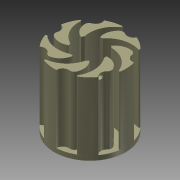
# Autodesk Inventor part: mecanum adapter
Saved by Autodesk Inventor 2015 (Build 190159000, 159)
## iProperties
Created: 2015-06-15
Part Number: mecanum adapter
Material: PBT Plastic
Document SubType Name: Modeling
Designer: Eduardo
Density: 1.31 g/cm^3
Appearance: Smooth - Ash
Author: Eduardo
Autodesk Inventor part; units mm, degrees
sketch "Sketch1" plane through (0, 0, 0) normal (0, 1, 0) x (-1, 0, 0)
  circle A0 centre (-2, -1.4) radius 8.6
  spline S0 degree 3 poles (5.001344, -1.681513) (4.992875, -1.892141) (4.974942, -2.101855) (4.947573, -2.310661) (4.933888, -2.415064) (4.917836, -2.519239) (4.89941, -2.623185) (4.880984, -2.727131) (4.858346, -2.840009) (4.833661, -2.948917) (4.734921, -3.384548) (4.597962, -3.804345) (4.410014, -4.230097) (4.222066, -4.655849) (3.994283, -5.059483) (3.719702, -5.447551) (3.445121, -5.83562) (3.130869, -6.195565) (2.783456, -6.52018) (2.522897, -6.76364) (2.245078, -6.986153) (1.949885, -7.187605) (1.851487, -7.254756) (1.752962, -7.318352) (1.653634, -7.379049) (1.355648, -7.561141) (1.045536, -7.720218) (0.723215, -7.856172) (0.669495, -7.878831) (0.613897, -7.901438) (0.561796, -7.921904) (0.171037, -8.075397) (-0.230384, -8.192863) (-0.642498, -8.274244) (-0.669972, -8.279669) (-0.699102, -8.285231) (-0.725059, -8.290035) (-0.776973, -8.299642) (-0.828947, -8.308653) (-0.88098, -8.317071) (-1.297249, -8.384413) (-1.719077, -8.414013) (-2.140737, -8.405573) (-2.351568, -8.401353) (-2.56161, -8.387632) (-2.770875, -8.364469) (-2.980139, -8.341306) (-3.18411, -8.309825) (-3.403209, -8.265052) (-3.622307, -8.220279) (-3.838521, -8.165183) (-4.051879, -8.099841) (-4.265237, -8.034498) (-4.472115, -7.96054) (-4.687338, -7.871176) (-4.902561, -7.781811) (-5.112501, -7.682071) (-5.31721, -7.572049) (-5.521919, -7.462027) (-5.719614, -7.342965) (-5.917021, -7.209885) (-6.311834, -6.943725) (-6.677588, -6.638718) (-7.010542, -6.298179) (-7.260258, -6.042774) (-7.488918, -5.770025) (-7.696638, -5.479998) (-7.765878, -5.383323) (-7.833557, -5.283445) (-7.896548, -5.185326) (-8.117015, -4.841909) (-8.306061, -4.481933) (-8.463671, -4.105364) (-8.486187, -4.051568) (-8.508354, -3.996632) (-8.528677, -3.944488) (-8.670936, -3.579483) (-8.781801, -3.20519) (-8.861277, -2.821592) (-8.872631, -2.766792) (-8.883729, -2.709613) (-8.8932, -2.657707) (-8.968967, -2.242459) (-9.006938, -1.82323) (-9.007002, -1.4) knots 0.01370505 0.01370505 0.01370505 0.01370505 0.04452677 0.04452677 0.04452677 0.05993763 0.05993763 0.05993763 0.07534849 0.07534849 0.07534849 0.13699192 0.13699192 0.13699192 0.19863536 0.19863536 0.19863536 0.26027879 0.26027879 0.26027879 0.30651137 0.30651137 0.30651137 0.32192222 0.32192222 0.32192222 0.3681548 0.3681548 0.3681548 0.37586023 0.37586023 0.37586023 0.43365095 0.43365095 0.43365095 0.43750366 0.43750366 0.43750366 0.44520909 0.44520909 0.44520909 0.50685253 0.50685253 0.50685253 0.53767424 0.53767424 0.53767424 0.56849596 0.56849596 0.56849596 0.59931768 0.59931768 0.59931768 0.63013939 0.63013939 0.63013939 0.66096111 0.66096111 0.66096111 0.69178283 0.69178283 0.69178283 0.75342626 0.75342626 0.75342626 0.79965884 0.79965884 0.79965884 0.8150697 0.8150697 0.8150697 0.8690077 0.8690077 0.8690077 0.87671313 0.87671313 0.87671313 0.93065114 0.93065114 0.93065114 0.93835657 0.93835657 0.93835657 1 1 1 1
  arc A1 (-18.018874, 4.997058) -> (-18.351886, 1.829471) centre (-16.268801, 3.211773) ccw
  arc A2 (-18.018874, 4.997058) -> (-18.337344, 10.272452) centre (-20.468977, 7.496458) ccw
  arc A3 (-12.372846, 15.791829) -> (-18.337344, 10.272452) centre (-2.000002, -1.400001) ccw
  spline S1 degree 3 poles (-12.372846, 15.791829) (-12.335731, 15.814222) (-12.295866, 15.831704) (-12.211456, 15.856299) (-12.167188, 15.862994) (-12.056492, 15.864827) (-11.990804, 15.852785) (-11.868157, 15.803892) (-11.812382, 15.767613) (-11.7181, 15.675458) (-11.680539, 15.620482) (-11.628788, 15.498824) (-11.615227, 15.433296) (-11.614528, 15.322052) (-11.620306, 15.277238) (-11.643312, 15.191649) (-11.660098, 15.151156) (-11.681913, 15.113352) knots 0 0 0 0 0.09833845 0.09833845 0.19946055 0.19946055 0.34950597 0.34950597 0.49900679 0.49900679 0.64861017 0.64861017 0.79894055 0.79894055 0.90098302 0.90098302 1 1 1 1
  arc A4 (-11.681591, 15.113908) -> (-10.569712, -0.678861) centre (0.574009, 8.041231) ccw
  arc A5 (-17.670798, 0.887063) -> (-10.564997, -2.176539) centre (-11.300504, 5.889999) ccw
  arc A6 (-18.351886, 1.829471) -> (-17.670798, 0.887063) centre (-6.219999, 9.879994) ccw
  circle A7 centre (-2, -1.4) radius 8.6
  arc A8 (-18.018874, 4.997058) -> (-18.337344, 10.272452) centre (-20.468977, 7.496458) ccw
  arc A9 (-12.372846, 15.791829) -> (-18.337344, 10.272452) centre (-1.999996, -1.400008) ccw
  arc A10 (-11.681913, 15.113352) -> (-12.372846, 15.791829) centre (-12.114582, 15.363786) ccw
  arc A11 (-11.681913, 15.113352) -> (-10.569712, -0.678861) centre (0.574009, 8.041231) ccw
  line L0 (-0.398255, -2.148255) -> (-0.398255, -0.651745)
  line L1 (-0.397937, -0.548255) -> (-0.397937, 0.201419)
  line L2 (-0.397937, 0.201419) -> (-1.148263, 0.201419)
  line L3 (-2.748263, 0.201737) -> (-1.251737, 0.201737)
  line L4 (-3.602063, 0.201419) -> (-2.851737, 0.201419)
  line L5 (-3.602063, -0.548255) -> (-3.602063, 0.201419)
  line L6 (-3.601745, -2.148255) -> (-3.601745, -0.651745)
  line L7 (-3.602063, -3.001419) -> (-3.602063, -2.251745)
  line L8 (-2.851737, -3.001419) -> (-3.602063, -3.001419)
  line L9 (-1.251737, -3.001737) -> (-2.748263, -3.001737)
  line L10 (-1.148263, -3.001419) -> (-0.397937, -3.001419)
  line L11 (-0.397937, -3.001419) -> (-0.397937, -2.251745)
  line L12 (-0.397937, -3.001419) -> (-3.602063, -3.001419)
  line L13 (-3.602063, -3.001419) -> (-3.602063, 0.201419)
  line L14 (-3.602063, 0.201419) -> (-0.397937, 0.201419)
  line L15 (-0.397937, 0.201419) -> (-0.397937, -3.001419)
  circle A12 centre (-2, -1.4) radius 7.006978
  arc A13 (-10.564997, -2.176539) -> (-10.569712, -0.678861) centre (-2.000683, -1.400733) ccw
  arc A14 (-10.564997, -2.176539) -> (-10.569712, -0.678861) centre (-2.000683, -1.400733) ccw
  arc A15 (-10.564997, -2.176539) -> (-10.569712, -0.678861) centre (-2.000693, -1.400733) ccw
  circle A16 centre (-2.000693, -1.400733) radius 8.599371
  arc A17 (-13.558681, -12.225962) -> (-6.733066, -8.580549) centre (-13.49832, -4.126187) ccw
  arc A18 (-20.947232, 1.326283) -> (-21.908476, 1.209113) centre (-21.412795, 1.144151) ccw
  spline S2 degree 3 poles (-21.908476, 1.209113) (-21.902844, 1.252092) (-21.891656, 1.294159) (-21.858257, 1.375488) (-21.835891, 1.414273) (-21.768306, 1.501961) (-21.717935, 1.545811) (-21.603239, 1.611216) (-21.540101, 1.632203) (-21.409268, 1.648458) (-21.342866, 1.643547) (-21.215484, 1.608155) (-21.155797, 1.577902) (-21.068388, 1.509089) (-21.036952, 1.476631) (-20.98438, 1.40528) (-20.963188, 1.366909) (-20.947232, 1.326283) knots 0 0 0 0 0.09833845 0.09833845 0.19946055 0.19946055 0.34950597 0.34950597 0.49900679 0.49900679 0.64861017 0.64861017 0.79894055 0.79894055 0.90098302 0.90098302 1 1 1 1
  arc A19 (-21.908476, 1.209113) -> (-21.312057, -6.895395) centre (-1.999991, -1.400002) ccw
  arc A20 (-21.908476, 1.209113) -> (-21.312057, -6.895395) centre (-2, -1.400002) ccw
  arc A21 (-20.947467, 1.32688) -> (-7.906937, -7.650447) centre (-7.776583, 6.498952) ccw
  arc A22 (-20.947232, 1.326283) -> (-7.906937, -7.650447) centre (-7.776583, 6.498953) ccw
  arc A23 (-16.989026, -9.93556) -> (-21.312057, -6.895395) centre (-20.470749, -10.292777) ccw
  arc A24 (-16.989026, -9.93556) -> (-21.312057, -6.895395) centre (-20.470749, -10.292777) ccw
  arc A25 (-16.989026, -9.93556) -> (-14.720136, -12.170877) centre (-14.502081, -9.680404) ccw
  arc A26 (-14.720136, -12.170877) -> (-13.558681, -12.225962) centre (-13.450181, 2.333633) ccw
  arc A27 (-0.742641, -17.186818) -> (0.662961, -9.577459) centre (-7.037666, -12.089499) ccw
  arc A28 (-15.9449, -14.513733) -> (-16.452618, -15.338318) centre (-16.092777, -14.991282) ccw
  spline S3 degree 3 poles (-16.452618, -15.338318) (-16.482709, -15.307117) (-16.508623, -15.272142) (-16.551385, -15.195322) (-16.567763, -15.153653) (-16.594181, -15.04614) (-16.597059, -14.979419) (-16.576683, -14.848968) (-16.553725, -14.786518) (-16.484861, -14.674094) (-16.43962, -14.625241) (-16.332528, -14.547717) (-16.271661, -14.519914) (-16.163362, -14.494479) (-16.118386, -14.490139) (-16.029823, -14.493523) (-15.986611, -14.500878) (-15.9449, -14.513733) knots 0 0 0 0 0.09833845 0.09833845 0.19946055 0.19946055 0.34950597 0.34950597 0.49900679 0.49900679 0.64861017 0.64861017 0.79894055 0.79894055 0.90098302 0.90098302 1 1 1 1
  arc A29 (-16.452618, -15.338318) -> (-9.744398, -19.925097) centre (-1.999993, -1.399994) ccw
  arc A30 (-16.452618, -15.338318) -> (-9.744398, -19.925097) centre (-1.999998, -1.400002) ccw
  arc A31 (-15.945513, -14.513544) -> (-0.796119, -9.91532) centre (-11.77729, -0.991398) ccw
  arc A32 (-15.9449, -14.513733) -> (-0.796119, -9.91532) centre (-11.777291, -0.991398) ccw
  arc A33 (-4.672136, -18.440727) -> (-9.744398, -19.925097) centre (-6.563671, -21.385569) ccw
  arc A34 (-4.672136, -18.440727) -> (-9.744398, -19.925097) centre (-6.563671, -21.385569) ccw
  arc A35 (-4.672136, -18.440727) -> (-1.509865, -18.060535) centre (-3.321039, -16.337268) ccw
  arc A36 (-1.509865, -18.060535) -> (-0.742641, -17.186818) centre (-12.058143, -8.024229) ccw
  arc A37 (11.126581, -10.259877) -> (6.053723, -4.416576) centre (3.216453, -12.003399) ccw
  arc A38 (-0.441773, -20.478841) -> (-0.113644, -21.389911) centre (-0.160611, -20.892202) ccw
  spline S4 degree 3 poles (-0.113644, -21.389911) (-0.156799, -21.393984) (-0.200301, -21.392438) (-0.287023, -21.377973) (-0.329813, -21.364798) (-0.430341, -21.31842) (-0.4843, -21.27907) (-0.573587, -21.181804) (-0.608098, -21.124918) (-0.653058, -21.000982) (-0.663046, -20.935153) (-0.656887, -20.803089) (-0.640674, -20.738166) (-0.593036, -20.637636) (-0.568387, -20.599767) (-0.510524, -20.532635) (-0.47783, -20.503436) (-0.441773, -20.478841) knots 0 0 0 0 0.09833845 0.09833845 0.19946055 0.19946055 0.34950597 0.34950597 0.49900679 0.49900679 0.64861017 0.64861017 0.79894055 0.79894055 0.90098302 0.90098302 1 1 1 1
  arc A39 (-0.113644, -21.389911) -> (7.654951, -19.005023) centre (-2, -1.399991) ccw
  arc A40 (-0.113644, -21.389911) -> (7.654951, -19.005023) centre (-1.999998, -1.4) ccw
  arc A41 (-0.442304, -20.479202) -> (5.408153, -5.767983) centre (-8.415498, -8.789434) ccw
  arc A42 (-0.441773, -20.478841) -> (5.408153, -5.767983) centre (-8.415499, -8.789435) ccw
  arc A43 (9.656927, -14.113879) -> (7.654951, -19.005023) centre (10.779945, -17.42882) ccw
  arc A44 (9.656927, -14.113879) -> (7.654951, -19.005023) centre (10.779945, -17.42882) ccw
  arc A45 (9.656927, -14.113879) -> (11.331325, -11.404471) centre (8.854772, -11.746064) ccw
  arc A46 (11.331325, -11.404471) -> (11.126581, -10.259877) centre (-3.092119, -13.393912) ccw
  arc A47 (13.11122, 3.338731) -> (5.379868, 3.01585) centre (9.542477, -3.932724) ccw
  arc A48 (13.887977, -12.077192) -> (14.804866, -12.388693) centre (14.386458, -12.115097) ccw
  spline S5 degree 3 poles (14.804866, -12.388693) (14.781143, -12.424972) (14.752811, -12.45802) (14.687432, -12.516803) (14.650453, -12.542043) (14.551514, -12.591723) (14.487106, -12.609375) (14.355391, -12.618538) (14.289399, -12.610053) (14.16447, -12.567931) (14.106775, -12.534696) (14.007363, -12.44754) (13.966714, -12.394385) (13.917817, -12.294462) (13.903578, -12.251579) (13.88717, -12.164484) (13.884725, -12.120718) (13.887977, -12.077192) knots 0 0 0 0 0.09833845 0.09833845 0.19946055 0.19946055 0.34950597 0.34950597 0.49900679 0.49900679 0.64861017 0.64861017 0.79894055 0.79894055 0.90098302 0.90098302 1 1 1 1
  arc A49 (14.804866, -12.388693) -> (17.783925, -4.828008) centre (-2.000007, -1.399995) ccw
  arc A50 (14.804866, -12.388693) -> (17.783925, -4.828008) centre (-1.999999, -1.399998) ccw
  arc A51 (13.887929, -12.077832) -> (6.033934, 1.668534) centre (-0.222705, -11.023076) ccw
  arc A52 (13.887977, -12.077192) -> (6.033934, 1.668534) centre (-0.222705, -11.023076) ccw
  arc A53 (15.208086, -0.213221) -> (17.783925, -4.828008) centre (18.500001, -1.402043) ccw
  arc A54 (15.208086, -0.213221) -> (17.783925, -4.828008) centre (18.500001, -1.402043) ccw
  arc A55 (15.208086, -0.213221) -> (14.133755, 2.785164) centre (12.856718, 0.635937) ccw
  arc A56 (14.133755, 2.785164) -> (13.11122, 3.338731) centre (6.696293, -9.731935) ccw
  arc A57 (3.716802, 13.368979) -> (-0.851178, 7.123051) centre (7.17678, 6.045144) ccw
  arc A58 (16.253756, 4.3646) -> (17.068969, 4.887235) centre (16.594189, 4.730695) ccw
  spline S6 degree 3 poles (17.068969, 4.887235) (17.082542, 4.846068) (17.090715, 4.803313) (17.09591, 4.715546) (17.092587, 4.670898) (17.069742, 4.56257) (17.043385, 4.501208) (16.968426, 4.392515) (16.920646, 4.346212) (16.809822, 4.2748) (16.747865, 4.250414) (16.617742, 4.227032) (16.55084, 4.228392) (16.44223, 4.252465) (16.399825, 4.268069) (16.321501, 4.309544) (16.285759, 4.33492) (16.253756, 4.3646) knots 0 0 0 0 0.09833845 0.09833845 0.19946055 0.19946055 0.34950597 0.34950597 0.49900679 0.49900679 0.64861017 0.64861017 0.79894055 0.79894055 0.90098302 0.90098302 1 1 1 1
  arc A59 (17.068969, 4.887235) -> (13.0152, 11.930368) centre (-2.000008, -1.400002) ccw
  arc A60 (17.068969, 4.887235) -> (13.0152, 11.930368) centre (-2.000001, -1.399998) ccw
  arc A61 (16.254227, 4.364163) -> (0.609999, 6.794382) centre (6.631749, -6.010345) ccw
  arc A62 (16.253756, 4.3646) -> (0.609999, 6.794382) centre (6.631749, -6.010345) ccw
  arc A63 (7.801205, 12.793768) -> (13.0152, 11.930368) centre (10.783139, 14.626273) ccw
  arc A64 (7.801205, 12.793768) -> (13.0152, 11.930368) centre (10.783139, 14.626273) ccw
  arc A65 (7.801205, 12.793768) -> (4.787139, 13.823285) centre (5.671253, 11.484836) ccw
  arc A66 (4.787139, 13.823285) -> (3.716802, 13.368979) centre (9.936219, 0.20416) ccw
  arc A67 (-9.982484, 12.277884) -> (-7.947311, 4.81222) centre (-2.099219, 10.416667) ccw
  arc A68 (4.874085, 16.465531) -> (4.97375, 17.428747) centre (4.800117, 16.959949) ccw
  spline S7 degree 3 poles (4.97375, 17.428747) (5.014398, 17.413692) (5.052921, 17.393424) (5.124779, 17.342765) (5.157614, 17.312329) (5.228065, 17.226926) (5.259607, 17.168061) (5.297849, 17.041687) (5.304261, 16.975461) (5.290995, 16.844291) (5.271431, 16.780647) (5.208581, 16.664334) (5.165805, 16.612876) (5.079267, 16.54297) (5.040628, 16.519546) (4.959367, 16.484169) (4.917243, 16.472046) (4.874085, 16.465531) knots 0 0 0 0 0.09833845 0.09833845 0.19946055 0.19946055 0.34950597 0.34950597 0.49900679 0.49900679 0.64861017 0.64861017 0.79894055 0.79894055 0.90098302 0.90098302 1 1 1 1
  arc A69 (4.97375, 17.428747) -> (-3.060277, 18.650704) centre (-2.000003, -1.400008) ccw
  arc A70 (4.97375, 17.428747) -> (-3.060277, 18.650704) centre (-2.000002, -1.399999) ccw
  arc A71 (4.87472, 16.465626) -> (-6.779318, 5.749693) centre (6.98632, 2.47407) ccw
  arc A72 (4.874085, 16.465531) -> (-6.779318, 5.749693) centre (6.98632, 2.47407) ccw
  arc A73 (-6.986183, 15.11256) -> (-3.060277, 18.650704) centre (-6.559688, 18.586478) ccw
  arc A74 (-6.986183, 15.11256) -> (-3.060277, 18.650704) centre (-6.559688, 18.586478) ccw
  arc A75 (-6.986183, 15.11256) -> (-9.670332, 13.397962) centre (-7.290823, 12.631191) ccw
  arc A76 (-9.670332, 13.397962) -> (-9.982484, 12.277884) centre (4.187928, 8.932289) ccw
  circle A77 centre (-2.000002, -1.399999) radius 8.600321
  arc A78 (-13.558681, -12.22596) -> (-6.733066, -8.580547) centre (-13.49832, -4.126185) ccw
  arc A79 (-20.947233, 1.326285) -> (-21.908477, 1.209115) centre (-21.412795, 1.144153) ccw
  spline S8 degree 3 poles (-21.908477, 1.209115) (-21.902844, 1.252094) (-21.891656, 1.294161) (-21.858257, 1.37549) (-21.835891, 1.414275) (-21.768306, 1.501963) (-21.717935, 1.545813) (-21.60324, 1.611217) (-21.540101, 1.632205) (-21.409268, 1.64846) (-21.342866, 1.643549) (-21.215484, 1.608156) (-21.155797, 1.577903) (-21.068388, 1.509091) (-21.036953, 1.476632) (-20.98438, 1.405282) (-20.963188, 1.366911) (-20.947233, 1.326285) knots 0 0 0 0 0.09833845 0.09833845 0.19946055 0.19946055 0.34950597 0.34950597 0.49900679 0.49900679 0.64861017 0.64861017 0.79894055 0.79894055 0.90098302 0.90098302 1 1 1 1
  arc A80 (-21.908477, 1.209115) -> (-21.312058, -6.895393) centre (-1.999992, -1.4) ccw
  arc A81 (-21.908477, 1.209115) -> (-21.312058, -6.895393) centre (-2, -1.4) ccw
  arc A82 (-20.947467, 1.326882) -> (-7.906938, -7.650445) centre (-7.776583, 6.498954) ccw
  arc A83 (-20.947233, 1.326285) -> (-7.906938, -7.650445) centre (-7.776584, 6.498955) ccw
  arc A84 (-16.989026, -9.935558) -> (-21.312058, -6.895393) centre (-20.470749, -10.292775) ccw
  arc A85 (-16.989026, -9.935558) -> (-21.312058, -6.895393) centre (-20.470749, -10.292775) ccw
  arc A86 (-16.989026, -9.935558) -> (-14.720137, -12.170875) centre (-14.502081, -9.680403) ccw
  arc A87 (-14.720137, -12.170875) -> (-13.558681, -12.22596) centre (-13.450181, 2.333635) ccw
  arc A88 (-17.670798, 0.887065) -> (-10.564997, -2.176537) centre (-11.300504, 5.890001) ccw
  arc A89 (-18.351886, 1.829473) -> (-17.670798, 0.887065) centre (-6.219999, 9.879996) ccw
  arc A90 (-0.742643, -17.186815) -> (0.662959, -9.577456) centre (-7.037668, -12.089496) ccw
  arc A91 (-15.944902, -14.51373) -> (-16.45262, -15.338315) centre (-16.092779, -14.991279) ccw
  spline S9 degree 3 poles (-16.45262, -15.338315) (-16.482711, -15.307115) (-16.508625, -15.272139) (-16.551386, -15.195319) (-16.567765, -15.15365) (-16.594183, -15.046137) (-16.597061, -14.979417) (-16.576685, -14.848965) (-16.553727, -14.786516) (-16.484862, -14.674091) (-16.439622, -14.625238) (-16.33253, -14.547714) (-16.271663, -14.519911) (-16.163364, -14.494476) (-16.118388, -14.490136) (-16.029825, -14.49352) (-15.986612, -14.500875) (-15.944902, -14.51373) knots 0 0 0 0 0.09833845 0.09833845 0.19946055 0.19946055 0.34950597 0.34950597 0.49900679 0.49900679 0.64861017 0.64861017 0.79894055 0.79894055 0.90098302 0.90098302 1 1 1 1
  arc A92 (-16.45262, -15.338315) -> (-9.7444, -19.925095) centre (-1.999995, -1.399991) ccw
  arc A93 (-16.45262, -15.338315) -> (-9.7444, -19.925095) centre (-2, -1.399999) ccw
  arc A94 (-15.945515, -14.513541) -> (-0.796121, -9.915317) centre (-11.777292, -0.991395) ccw
  arc A95 (-15.944902, -14.51373) -> (-0.796121, -9.915317) centre (-11.777293, -0.991395) ccw
  arc A96 (-4.672137, -18.440724) -> (-9.7444, -19.925095) centre (-6.563673, -21.385566) ccw
  arc A97 (-4.672137, -18.440724) -> (-9.7444, -19.925095) centre (-6.563673, -21.385566) ccw
  arc A98 (-4.672137, -18.440724) -> (-1.509867, -18.060532) centre (-3.321041, -16.337265) ccw
  arc A99 (-1.509867, -18.060532) -> (-0.742643, -17.186815) centre (-12.058145, -8.024226) ccw
  arc A100 (-13.558682, -12.225959) -> (-6.733068, -8.580546) centre (-13.498322, -4.126184) ccw
  arc A101 (-14.720138, -12.170874) -> (-13.558682, -12.225959) centre (-13.450182, 2.333636) ccw
  arc A102 (11.126578, -10.259875) -> (6.05372, -4.416573) centre (3.216449, -12.003397) ccw
  arc A103 (-0.441777, -20.478838) -> (-0.113648, -21.389909) centre (-0.160614, -20.8922) ccw
  spline S10 degree 3 poles (-0.113648, -21.389909) (-0.156803, -21.393981) (-0.200305, -21.392435) (-0.287027, -21.377971) (-0.329816, -21.364796) (-0.430345, -21.318418) (-0.484303, -21.279068) (-0.573591, -21.181801) (-0.608101, -21.124916) (-0.653062, -21.00098) (-0.66305, -20.93515) (-0.65689, -20.803087) (-0.640677, -20.738164) (-0.59304, -20.637634) (-0.568391, -20.599764) (-0.510527, -20.532633) (-0.477834, -20.503434) (-0.441777, -20.478838) knots 0 0 0 0 0.09833845 0.09833845 0.19946055 0.19946055 0.34950597 0.34950597 0.49900679 0.49900679 0.64861017 0.64861017 0.79894055 0.79894055 0.90098302 0.90098302 1 1 1 1
  arc A104 (-0.113648, -21.389909) -> (7.654948, -19.005021) centre (-2.000004, -1.399989) ccw
  arc A105 (-0.113648, -21.389909) -> (7.654948, -19.005021) centre (-2.000001, -1.399997) ccw
  arc A106 (-0.442308, -20.4792) -> (5.408149, -5.76798) centre (-8.415502, -8.789432) ccw
  arc A107 (-0.441777, -20.478838) -> (5.408149, -5.76798) centre (-8.415502, -8.789432) ccw
  arc A108 (9.656924, -14.113877) -> (7.654948, -19.005021) centre (10.779941, -17.428817) ccw
  arc A109 (9.656924, -14.113877) -> (7.654948, -19.005021) centre (10.779941, -17.428817) ccw
  arc A110 (9.656924, -14.113877) -> (11.331321, -11.404468) centre (8.854769, -11.746062) ccw
  arc A111 (11.331321, -11.404468) -> (11.126578, -10.259875) centre (-3.092122, -13.39391) ccw
  arc A112 (-0.742645, -17.186815) -> (0.662957, -9.577456) centre (-7.03767, -12.089496) ccw
  arc A113 (-1.509869, -18.060533) -> (-0.742645, -17.186815) centre (-12.058147, -8.024227) ccw
  arc A114 (13.111216, 3.338732) -> (5.379864, 3.015851) centre (9.542472, -3.932724) ccw
  arc A115 (13.887972, -12.077191) -> (14.804861, -12.388693) centre (14.386454, -12.115096) ccw
  spline S11 degree 3 poles (14.804861, -12.388693) (14.781139, -12.424972) (14.752807, -12.458019) (14.687428, -12.516803) (14.650448, -12.542042) (14.55151, -12.591722) (14.487102, -12.609375) (14.355387, -12.618538) (14.289395, -12.610052) (14.164465, -12.567931) (14.10677, -12.534695) (14.007359, -12.447539) (13.966709, -12.394385) (13.917813, -12.294461) (13.903574, -12.251578) (13.887166, -12.164483) (13.884721, -12.120717) (13.887972, -12.077191) knots 0 0 0 0 0.09833845 0.09833845 0.19946055 0.19946055 0.34950597 0.34950597 0.49900679 0.49900679 0.64861017 0.64861017 0.79894055 0.79894055 0.90098302 0.90098302 1 1 1 1
  arc A116 (14.804861, -12.388693) -> (17.783921, -4.828007) centre (-2.000011, -1.399994) ccw
  arc A117 (14.804861, -12.388693) -> (17.783921, -4.828007) centre (-2.000003, -1.399998) ccw
  arc A118 (13.887924, -12.077832) -> (6.03393, 1.668535) centre (-0.22271, -11.023075) ccw
  arc A119 (13.887972, -12.077191) -> (6.03393, 1.668535) centre (-0.22271, -11.023075) ccw
  arc A120 (15.208082, -0.213221) -> (17.783921, -4.828007) centre (18.499997, -1.402042) ccw
  arc A121 (15.208082, -0.213221) -> (17.783921, -4.828007) centre (18.499997, -1.402042) ccw
  arc A122 (15.208082, -0.213221) -> (14.133751, 2.785165) centre (12.856714, 0.635938) ccw
  arc A123 (14.133751, 2.785165) -> (13.111216, 3.338732) centre (6.696289, -9.731934) ccw
  arc A124 (11.126577, -10.259877) -> (6.053719, -4.416575) centre (3.216449, -12.003399) ccw
  arc A125 (11.331321, -11.40447) -> (11.126577, -10.259877) centre (-3.092123, -13.393912) ccw
  arc A126 (3.716799, 13.368978) -> (-0.851182, 7.12305) centre (7.176777, 6.045143) ccw
  arc A127 (16.253753, 4.364599) -> (17.068966, 4.887234) centre (16.594186, 4.730694) ccw
  spline S12 degree 3 poles (17.068966, 4.887234) (17.082539, 4.846067) (17.090712, 4.803311) (17.095907, 4.715545) (17.092584, 4.670897) (17.069738, 4.562569) (17.043382, 4.501207) (16.968423, 4.392514) (16.920643, 4.346211) (16.809819, 4.274799) (16.747862, 4.250413) (16.617739, 4.227031) (16.550836, 4.228391) (16.442226, 4.252464) (16.399821, 4.268068) (16.321497, 4.309543) (16.285755, 4.334919) (16.253753, 4.364599) knots 0 0 0 0 0.09833845 0.09833845 0.19946055 0.19946055 0.34950597 0.34950597 0.49900679 0.49900679 0.64861017 0.64861017 0.79894055 0.79894055 0.90098302 0.90098302 1 1 1 1
  arc A128 (17.068966, 4.887234) -> (13.015197, 11.930367) centre (-2.000012, -1.400003) ccw
  arc A129 (17.068966, 4.887234) -> (13.015197, 11.930367) centre (-2.000004, -1.399999) ccw
  arc A130 (16.254223, 4.364162) -> (0.609996, 6.794381) centre (6.631745, -6.010346) ccw
  arc A131 (16.253753, 4.364599) -> (0.609996, 6.794381) centre (6.631746, -6.010346) ccw
  arc A132 (7.801202, 12.793767) -> (13.015197, 11.930367) centre (10.783135, 14.626272) ccw
  arc A133 (7.801202, 12.793767) -> (13.015197, 11.930367) centre (10.783135, 14.626272) ccw
  arc A134 (7.801202, 12.793767) -> (4.787135, 13.823284) centre (5.671249, 11.484835) ccw
  arc A135 (4.787135, 13.823284) -> (3.716799, 13.368978) centre (9.936216, 0.204159) ccw
  arc A136 (13.111217, 3.33873) -> (5.379865, 3.015849) centre (9.542473, -3.932725) ccw
  arc A137 (14.133752, 2.785163) -> (13.111217, 3.33873) centre (6.69629, -9.731936) ccw
  arc A138 (-9.982486, 12.277882) -> (-7.947312, 4.812219) centre (-2.099221, 10.416666) ccw
  arc A139 (4.874084, 16.465529) -> (4.973748, 17.428746) centre (4.800116, 16.959947) ccw
  spline S13 degree 3 poles (4.973748, 17.428746) (5.014396, 17.41369) (5.05292, 17.393423) (5.124777, 17.342763) (5.157613, 17.312328) (5.228063, 17.226924) (5.259605, 17.168059) (5.297848, 17.041685) (5.304259, 16.97546) (5.290993, 16.84429) (5.27143, 16.780646) (5.20858, 16.664333) (5.165804, 16.612874) (5.079266, 16.542969) (5.040626, 16.519544) (4.959366, 16.484167) (4.917241, 16.472045) (4.874084, 16.465529) knots 0 0 0 0 0.09833845 0.09833845 0.19946055 0.19946055 0.34950597 0.34950597 0.49900679 0.49900679 0.64861017 0.64861017 0.79894055 0.79894055 0.90098302 0.90098302 1 1 1 1
  arc A140 (4.973748, 17.428746) -> (-3.060279, 18.650703) centre (-2.000005, -1.400009) ccw
  arc A141 (4.973748, 17.428746) -> (-3.060279, 18.650703) centre (-2.000003, -1.400001) ccw
  arc A142 (4.874719, 16.465625) -> (-6.77932, 5.749692) centre (6.986318, 2.474069) ccw
  arc A143 (4.874084, 16.465529) -> (-6.77932, 5.749692) centre (6.986319, 2.474069) ccw
  arc A144 (-6.986185, 15.112559) -> (-3.060279, 18.650703) centre (-6.559689, 18.586476) ccw
  arc A145 (-6.986185, 15.112559) -> (-3.060279, 18.650703) centre (-6.559689, 18.586476) ccw
  arc A146 (-6.986185, 15.112559) -> (-9.670333, 13.39796) centre (-7.290824, 12.63119) ccw
  arc A147 (-9.670333, 13.39796) -> (-9.982486, 12.277882) centre (4.187927, 8.932288) ccw
  arc A148 (3.716801, 13.368977) -> (-0.85118, 7.12305) centre (7.176779, 6.045143) ccw
  arc A149 (4.787137, 13.823284) -> (3.716801, 13.368977) centre (9.936218, 0.204158) ccw
  arc A150 (5.379865, 3.015849) -> (6.033931, 1.668533) centre (-2.000696, -1.399525) ccw
  arc A151 (-0.85118, 7.12305) -> (0.609998, 6.794381) centre (-2.001653, -1.404013) ccw
  arc A152 (-10.564997, -2.176537) -> (-10.569712, -0.678859) centre (-1.997207, -1.40072) ccw
  arc A153 (-6.733068, -8.580546) -> (-7.906939, -7.650444) centre (-1.99652, -1.39678) ccw
  arc A154 (0.662957, -9.577456) -> (-0.796122, -9.915317) centre (-2.004427, -1.377656) ccw
  arc A155 (6.053719, -4.416575) -> (5.408148, -5.767982) centre (-2.26403, -1.273064) ccw
  point P0 (0, 0)
  point P1 (5.38009, 3.015232)
  point P2 (-2, -1.4)
  point P3 (6.034164, 1.667933)
  point P4 (-2, -1.4)
  point P5 (-2, -1.4)
  point P6 (-2, -1.4)
  point P7 (-2, -1.4)
  point P8 (-2, -1.4)
  point P9 (-2, -1.4)
  point P10 (-2, -1.4)
  point P11 (-2, -1.4)
  point P12 (-2, -1.4)
  point P13 (-2, -1.4)
  point P14 (-2, -1.4)
  point P15 (-2, -1.4)
  point P16 (-2, -1.4)
  point P17 (-2, -1.4)
  point P18 (-2, -1.4)
  point P19 (-2, -1.4)
  point P20 (-2, -1.4)
  point P21 (-2, -1.4)
  point P22 (-2, -1.4)
  point P23 (-2, -1.4)
  point P24 (-2, -1.4)
  point P25 (-2, -1.4)
  point P26 (-2, -1.4)
  point P27 (-2, -1.4)
  point P28 (-2, -1.4)
  point P29 (-2, -1.4)
  point P30 (-2, -1.4)
  point P31 (-2, -1.4)
  point P32 (-2, -1.4)
  point P33 (-2, -1.4)
  point P34 (-2, -1.4)
  point P35 (-2, -1.4)
  point P36 (-2, -1.4)
  point P37 (-2, -1.4)
  point P38 (-2, -1.4)
  point P39 (-2, -1.4)
  point P40 (-2, -1.4)
  point P41 (-2, -1.4)
  point P42 (-2, -1.4)
  point P43 (-2, -1.4)
  point P44 (-2, -1.4)
  point P45 (-2, -1.4)
  point P46 (-2, -1.4)
  point P47 (-2, -1.4)
  point P48 (-2, -1.4)
  point P49 (-2, -1.4)
  point P50 (-2, -1.4)
  point P51 (-2, -1.4)
  point P52 (-2, -1.4)
  point P53 (6.053303, -4.417335)
  point P54 (-2, -1.4)
  point P55 (5.407717, -5.768722)
  point P56 (-2, -1.4)
  point P57 (-2, -1.4)
  point P58 (-2, -1.4)
  point P59 (-2, -1.4)
  point P60 (-2, -1.4)
  point P61 (-2, -1.4)
  point P62 (-2, -1.4)
  point P63 (-2, -1.4)
  point P64 (-2, -1.4)
  point P65 (-2, -1.4)
  point P66 (-2, -1.4)
  point P67 (-2, -1.4)
  point P68 (-2, -1.4)
  point P69 (-2, -1.4)
  point P70 (0.661901, -9.57767)
  point P71 (-0.79718, -9.91547)
  point P72 (-11.77724, -0.99018)
  point P73 (-2, -1.4)
  point P74 (-6.734071, -8.579733)
  point P75 (-13.498727, -4.124464)
  point P76 (-13.449627, 2.335349)
  point P77 (-2, -1.4)
  point P78 (-2, -1.4)
  point P79 (0.610408, 6.794252)
  point P80 (-2, -1.4)
  point P81 (-11.77724, -0.99018)
  point P82 (-13.498733, -4.124461)
  point P83 (-13.444614, 2.440039)
  point P84 (-2.000001, -1.4)
  point P85 (-1.999957, -1.39972)
  point P86 (-2.01143, -1.406578)
  point P87 (-6.368794, -6.878294)
  point P88 (-8.416419, -8.788635)
  point P89 (-7.039267, -12.088743)
  point P90 (-8.416419, -8.788635)
  point P91 (-7.039273, -12.088745)
  point P92 (-12.059139, -8.022727)
  point P93 (-12.137863, -7.953535)
  point P94 (-0.440796, -8.231322)
  point P95 (-0.223905, -11.023297)
  point P96 (3.214864, -12.00418)
  point P97 (-0.223905, -11.023297)
  point P98 (3.214862, -12.004186)
  point P99 (-3.093914, -13.393755)
  point P100 (-3.197095, -13.412163)
  point P101 (4.31309, -4.440224)
  point P102 (6.631174, -6.01142)
  point P103 (9.542096, -3.934453)
  point P104 (6.631174, -6.01142)
  point P105 (9.542099, -3.934459)
  point P106 (6.695051, -9.73324)
  point P107 (6.645111, -9.825387)
  point P108 (4.31309, 1.640224)
  point P109 (6.986803, 2.47295)
  point P110 (7.177895, 6.043768)
  point P111 (6.986803, 2.47295)
  point P112 (7.177901, 6.043768)
  point P113 (9.936465, 0.202374)
  point P114 (9.977371, 0.105877)
  point P115 (-0.440795, 5.431321)
  point P116 (0.575186, 8.04091)
  point P117 (-2.097449, 10.416681)
  point P118 (0.575186, 8.04091)
  point P119 (-2.097444, 10.416685)
  point P120 (4.189478, 8.931368)
  point P121 (4.290427, 8.903185)
  point P122 (-6.368794, 4.078295)
  point P123 (-7.775599, 6.499672)
  point P124 (-11.299411, 5.891391)
  point P125 (-7.775599, 6.499672)
  point P126 (-11.299412, 5.891398)
  point P127 (-6.218312, 9.880631)
  point P128 (-6.133337, 9.941985)
  point P129 (-6.368794, -6.878292)
  point P130 (-8.41642, -8.788633)
  point P131 (-8.41642, -8.788633)
  point P132 (-12.05914, -8.022725)
  point P133 (-12.137864, -7.953533)
  point P134 (-11.777291, -0.991397)
  point P135 (-11.777291, -0.991396)
  point P136 (-12.058143, -8.024227)
  point P137 (-8.415499, -8.789433)
  point P138 (-8.415499, -8.789433)
  point P139 (-13.498728, -4.124462)
  point P140 (-13.498733, -4.124459)
  point P141 (-9.007002, -1.399998)
  point P142 (-11.77724, -0.990178)
  point P143 (-11.77724, -0.990178)
  point P144 (-0.440798, -8.231319)
  point P145 (-0.223906, -11.023294)
  point P146 (-0.223906, -11.023294)
  point P147 (-3.093916, -13.393752)
  point P148 (-3.197096, -13.41216)
  point P149 (-8.4155, -8.789432)
  point P150 (-8.4155, -8.789431)
  point P151 (-3.09212, -13.393909)
  point P152 (-0.222707, -11.023073)
  point P153 (-0.222707, -11.023073)
  point P154 (-7.039269, -12.08874)
  point P155 (-7.039275, -12.088742)
  point P156 (-6.368796, -6.878291)
  point P157 (-8.416421, -8.788632)
  point P158 (-8.416421, -8.788632)
  point P159 (4.313087, -4.440222)
  point P160 (6.63117, -6.011418)
  point P161 (6.63117, -6.011418)
  point P162 (6.695047, -9.733238)
  point P163 (6.645107, -9.825385)
  point P164 (-0.222709, -11.023074)
  point P165 (-0.222709, -11.023073)
  point P166 (6.69629, -9.731932)
  point P167 (6.631745, -6.010342)
  point P168 (6.631745, -6.010342)
  point P169 (3.21486, -12.004178)
  point P170 (3.214858, -12.004184)
  point P171 (-0.440799, -8.231319)
  point P172 (-0.223908, -11.023295)
  point P173 (-0.223908, -11.023295)
  point P174 (4.313086, 1.640224)
  point P175 (6.986798, 2.472951)
  point P176 (6.986798, 2.472951)
  point P177 (9.936461, 0.202375)
  point P178 (9.977367, 0.105877)
  point P179 (6.631745, -6.010344)
  point P180 (6.631744, -6.010344)
  point P181 (9.936215, 0.20416)
  point P182 (6.986316, 2.474071)
  point P183 (6.986315, 2.47407)
  point P184 (9.542092, -3.934453)
  point P185 (9.542095, -3.934458)
  point P186 (4.313086, -4.440224)
  point P187 (6.63117, -6.01142)
  point P188 (6.63117, -6.01142)
  point P189 (-0.440798, 5.43132)
  point P190 (0.575182, 8.040909)
  point P191 (0.575182, 8.040909)
  point P192 (4.189474, 8.931367)
  point P193 (4.290424, 8.903184)
  point P194 (6.986317, 2.474069)
  point P195 (6.986316, 2.474069)
  point P196 (4.187925, 8.932288)
  point P197 (0.574006, 8.04123)
  point P198 (0.574006, 8.04123)
  point P199 (7.177891, 6.043767)
  dimension "d2" = 360
  dimension "d6" = 360
  constraints: 315 point on circle, 154 centre point, 32 end point, 5 tangent, 4 coincident, 2 perpendicular, 1 concentric, 1 horizontal, 1 vertical, 667 other
sketch "Sketch1 outline for Extrusion1" plane through (0, 0, 0) normal (0, 1, 0) x (-1, 0, 0)
  arc A0 (-17.670798, 0.887063) -> (-10.564997, -2.176539) centre (-11.300504, 5.889999) ccw
  arc A1 (-18.351886, 1.829471) -> (-17.670798, 0.887063) centre (-6.219999, 9.879994) ccw
  arc A2 (-18.018874, 4.997058) -> (-18.351886, 1.829471) centre (-16.268801, 3.211773) ccw
  arc A3 (-18.337344, 10.272452) -> (-18.018874, 4.997058) centre (-20.468977, 7.496458) cw
  arc A4 (-12.372846, 15.791829) -> (-18.337344, 10.272452) centre (-1.999996, -1.400008) ccw
  spline S0 degree 3 poles (-12.372846, 15.791829) (-12.335731, 15.814222) (-12.295866, 15.831704) (-12.211456, 15.856299) (-12.167188, 15.862994) (-12.056492, 15.864827) (-11.990804, 15.852785) (-11.868157, 15.803892) (-11.812382, 15.767613) (-11.7181, 15.675458) (-11.680539, 15.620482) (-11.628788, 15.498824) (-11.615227, 15.433296) (-11.614528, 15.322052) (-11.620306, 15.277238) (-11.643312, 15.191649) (-11.660098, 15.151156) (-11.681913, 15.113352) knots 0 0 0 0 0.09833845 0.09833845 0.19946055 0.19946055 0.34950597 0.34950597 0.49900679 0.49900679 0.64861017 0.64861017 0.79894055 0.79894055 0.90098302 0.90098302 1 1 1 1
  arc A5 (-10.569712, -0.678861) -> (-11.681913, 15.113352) centre (0.57401, 8.041231) cw
  arc A6 (-10.569712, -0.678861) -> (-10.564997, -2.176539) centre (-2.000693, -1.400733) ccw
extrude "Extrusion1" add sketch "Sketch1 outline for Extrusion1" along normal blind 38.1
ref_plane "Work Plane1" through (17.670798, 38.1, 0.887063) normal (0, 1, 0) x (1, 0, 0)
sketch "Sketch2" plane through (17.670798, 38.1, 0.887063) normal (0, 1, 0) x (1, 0, 0)
  circle A0 centre (-15.670798, 2.287063) radius 8.6
  circle A1 centre (-15.670798, 2.287063) radius 7.006978
  line L0 (-14.069052, 3.035318) -> (-14.069052, 1.538809)
  line L1 (-14.068735, 3.888483) -> (-14.068735, 3.138809)
  line L2 (-14.819061, 3.888483) -> (-14.068735, 3.888483)
  line L3 (-17.272861, 3.888483) -> (-14.068735, 3.888483)
  line L4 (-17.272861, 3.888483) -> (-17.272861, 3.138809)
  line L5 (-17.272543, 3.035318) -> (-17.272543, 1.538809)
  line L6 (-17.272861, 1.435318) -> (-17.272861, 0.685644)
  line L7 (-17.272861, 0.685644) -> (-17.272861, 3.888483)
  line L8 (-14.068735, 0.685644) -> (-17.272861, 0.685644)
  line L9 (-14.068735, 3.888483) -> (-14.068735, 0.685644)
  arc A2 (0, 0) -> (-7.105801, 3.063602) centre (-6.370293, -5.002935) ccw
  arc A3 (-5.988885, -14.226289) -> (-7.101086, 1.565924) centre (-18.244807, -7.154167) ccw
  arc A4 (0.348076, -4.109995) -> (0.681088, -0.942408) centre (-1.401997, -2.324709) ccw
  arc A5 (0.681088, -0.942408) -> (0, 0) centre (-11.450799, -8.992931) ccw
  arc A6 (0.348076, -4.109995) -> (0.666546, -9.385388) centre (2.798179, -6.609394) ccw
  arc A7 (-5.297952, -14.904765) -> (0.666546, -9.385388) centre (-15.670802, 2.287071) ccw
  arc A8 (0.681088, -0.942408) -> (-7.105801, 3.063602) centre (-6.364495, -5.066534) ccw
  arc A9 (0.348076, -4.109995) -> (0.681088, -0.942408) centre (-1.401997, -2.324709) ccw
  arc A10 (0.348076, -4.109995) -> (0.666546, -9.385388) centre (2.798179, -6.609394) ccw
  arc A11 (-5.297952, -14.904765) -> (0.666546, -9.385388) centre (-15.670802, 2.287071) ccw
  arc A12 (-5.988885, -14.226289) -> (-5.297952, -14.904765) centre (-5.556215, -14.476723) ccw
  arc A13 (-5.988885, -14.226289) -> (-7.101086, 1.565924) centre (-18.244807, -7.154168) ccw
  arc A14 (-7.101086, 1.565924) -> (-7.105801, 3.063602) centre (-15.670105, 2.287796) ccw
  circle A15 centre (-15.670105, 2.287796) radius 8.599371
  line L10 (-17.272861, 3.888483) -> (-14.068735, 3.888483)
  line L11 (-14.068735, 3.888483) -> (-14.068735, 0.685644)
  line L12 (-14.068735, 0.685644) -> (-17.272861, 0.685644)
  line L13 (-17.272861, 0.685644) -> (-17.272861, 3.888483)
  arc A16 (-2.949827, 13.057674) -> (-10.936898, 9.467346) centre (-4.118305, 4.977866) ccw
  arc A17 (-0.680938, 10.822357) -> (-2.949827, 13.057674) centre (-3.167883, 10.567202) ccw
  arc A18 (-0.680938, 10.822357) -> (3.642094, 7.782193) centre (2.800785, 11.179574) ccw
  arc A19 (4.238513, -0.322315) -> (3.642094, 7.782193) centre (-15.669972, 2.286799) ccw
  arc A20 (3.277269, -0.439485) -> (4.238513, -0.322315) centre (3.742831, -0.257353) ccw
  arc A21 (3.277269, -0.439485) -> (-9.763026, 8.537245) centre (-9.893381, -5.612155) ccw
  arc A22 (-9.763026, 8.537245) -> (-10.936898, 9.467346) centre (-15.670105, 2.287796) ccw
  circle A23 centre (-15.670105, 2.287796) radius 8.599371
  arc A24 (-16.159371, 18.947819) -> (-18.332197, 10.464743) centre (-10.570856, 12.996588) ccw
  arc A25 (-12.9971, 19.328011) -> (-16.159371, 18.947819) centre (-14.348197, 17.224552) ccw
  arc A26 (-12.9971, 19.328011) -> (-7.924838, 20.812382) centre (-11.105565, 22.272853) ccw
  arc A27 (-1.216617, 16.225602) -> (-7.924838, 20.812382) centre (-15.669242, 2.287278) ccw
  arc A28 (-1.724336, 15.401017) -> (-1.216617, 16.225602) centre (-1.576459, 15.878566) ccw
  arc A29 (-1.724336, 15.401017) -> (-16.873117, 10.802604) centre (-5.891945, 1.878682) ccw
  arc A30 (-16.873117, 10.802604) -> (-18.332197, 10.464743) centre (-15.670105, 2.287796) ccw
  circle A31 centre (-15.670105, 2.287796) radius 8.599371
  arc A32 (-29.000487, 12.292627) -> (-23.722886, 5.304732) centre (-20.863246, 12.951372) ccw
  arc A33 (-27.32609, 15.002035) -> (-29.000487, 12.292627) centre (-26.523935, 12.634221) ccw
  arc A34 (-27.32609, 15.002035) -> (-25.324114, 19.89318) centre (-28.449107, 18.316976) ccw
  arc A35 (-17.555518, 22.278068) -> (-25.324114, 19.89318) centre (-15.669162, 2.288148) ccw
  arc A36 (-17.227389, 21.366997) -> (-17.555518, 22.278068) centre (-17.508552, 21.780359) ccw
  arc A37 (-17.227389, 21.366997) -> (-23.077315, 6.656139) centre (-9.253663, 9.677591) ccw
  arc A38 (-23.077315, 6.656139) -> (-23.722886, 5.304732) centre (-15.670105, 2.287796) ccw
  circle A39 centre (-15.670105, 2.287796) radius 8.599371
  arc A40 (-31.803554, -1.896407) -> (-23.049667, -2.127093) centre (-27.245094, 4.876266) ccw
  arc A41 (-32.877885, 1.101979) -> (-31.803554, -1.896407) centre (-30.526517, 0.252821) ccw
  arc A42 (-32.877885, 1.101979) -> (-35.453724, 5.716765) centre (-36.1698, 2.2908) ccw
  arc A43 (-32.474664, 13.277451) -> (-35.453724, 5.716765) centre (-15.669792, 2.288753) ccw
  arc A44 (-31.557775, 12.96595) -> (-32.474664, 13.277451) centre (-32.056257, 13.003854) ccw
  arc A45 (-31.557775, 12.96595) -> (-23.703733, -0.779777) centre (-17.447093, 11.911834) ccw
  arc A46 (-23.703733, -0.779777) -> (-23.049667, -2.127093) centre (-15.670105, 2.287796) ccw
  circle A47 centre (-15.670105, 2.287796) radius 8.599371
  arc A48 (-22.457804, -12.93465) -> (-16.819487, -6.234416) centre (-24.91074, -5.14801) ccw
  arc A49 (-25.471871, -11.905133) -> (-22.457804, -12.93465) centre (-23.341918, -10.596201) ccw
  arc A50 (-25.471871, -11.905133) -> (-30.685865, -11.041733) centre (-28.453804, -13.737638) ccw
  arc A51 (-34.739634, -3.9986) -> (-30.685865, -11.041733) centre (-15.670657, 2.288637) ccw
  arc A52 (-33.924422, -3.475965) -> (-34.739634, -3.9986) centre (-34.264855, -3.84206) ccw
  arc A53 (-33.924422, -3.475965) -> (-18.280665, -5.905747) centre (-24.302414, 6.898981) ccw
  arc A54 (-18.280665, -5.905747) -> (-16.819487, -6.234416) centre (-15.670105, 2.287796) ccw
  circle A55 centre (-15.670105, 2.287796) radius 8.599371
  arc A56 (-8.000778, -12.510081) -> (-9.723799, -3.924339) centre (-15.617999, -9.572973) ccw
  arc A57 (-10.684927, -14.224679) -> (-8.000778, -12.510081) centre (-10.380287, -11.74331) ccw
  arc A58 (-10.684927, -14.224679) -> (-14.610833, -17.762823) centre (-11.111422, -17.698597) ccw
  arc A59 (-22.64486, -16.540866) -> (-14.610833, -17.762823) centre (-15.671107, 2.287889) ccw
  arc A60 (-22.545195, -15.57765) -> (-22.64486, -16.540866) centre (-22.471227, -16.072067) ccw
  arc A61 (-22.545195, -15.57765) -> (-10.891792, -4.861812) centre (-24.657431, -1.586189) ccw
  arc A62 (-10.891792, -4.861812) -> (-9.723799, -3.924339) centre (-15.670105, 2.287796) ccw
  circle A63 centre (-15.670105, 2.287796) radius 8.599371
  point P0 (-17.670798, 0.887063)
  point P1 (-4.111283, 13.11276)
  point P2 (-4.171644, 5.012985)
  point P3 (-3.167883, 10.567202)
  point P4 (2.800785, 11.179574)
  point P5 (-16.926595, 18.074102)
  point P6 (-10.63157, 12.976783)
  point P7 (-14.348197, 17.224552)
  point P8 (-28.795744, 11.148034)
  point P9 (-20.885615, 12.891556)
  point P10 (-26.523935, 12.634221)
  point P11 (-28.449107, 18.316976)
  point P12 (-30.781019, -2.449974)
  point P13 (-27.212275, 4.821482)
  point P14 (-30.526517, 0.252821)
  point P15 (-21.387468, -12.480343)
  point P16 (-24.847445, -5.156509)
  point P17 (-7.688626, -11.390003)
  point P18 (-15.571891, -9.528786)
  dimension "d12" = 360
  constraints: 98 point on circle, 56 centre point, 9 coincident, 8 end point, 4 tangent, 2 concentric, 2 perpendicular, 1 collinear, 1 horizontal, 190 other
extrude "Extrusion2" add sketch "Sketch2" against normal blind 38.1 contours A0 A16 A17 A18 A19 A20 A21 | A56 A57 A58 A59 A60 A61 A0 | A0 A24 A25 A26 A27 A28 A29 | A48 A49 A50 A51 A52 A53 A0 | A0 A32 A33 A34 A35 A36 A37 | A40 A41 A42 A43 A44 A45 A0
ref_plane "Work Plane2" through (18.458228, 0, -7.429575) normal (0, -1, 0) x (1, 0, 0)
sketch "Sketch3" plane through (18.458228, 0, -7.429575) normal (0, -1, 0) x (1, 0, 0)
  line L0 (-14.856165, 4.428156) -> (-14.856165, 7.630994)
  line L1 (-18.060291, 7.630994) -> (-18.060291, 4.428156)
  line L2 (-18.060291, 4.428156) -> (-14.856165, 4.428156)
  line L3 (-14.856165, 7.630994) -> (-18.060291, 7.630994)
  circle A0 centre (-16.458228, 6.029575) radius 8.6
  circle A1 centre (-16.458228, 6.029575) radius 20.079652
  line L4 (-14.856165, 7.630994) -> (-14.856165, 4.428156)
  line L5 (-14.856165, 4.428156) -> (-18.060291, 4.428156)
  line L6 (-18.060291, 4.428156) -> (-18.060291, 7.630994)
  line L7 (-18.060291, 7.630994) -> (-14.856165, 7.630994)
  point P0 (-18.458228, 7.429575)
  constraints: 8 end point, 3 collinear, 1 centre point, 1 coincident, 1 perpendicular
extrude "Extrusion3" add sketch "Sketch3" along normal blind 2.54 contours A0 | A1
sketch "Sketch5" plane through (2, -2.54, -1.4) normal (0, -1, 0) x (1, 0, 0)
  circle A0 centre (0, 0) radius 2.3622
  point P0 (-2, 1.4)
  dimension "d26" = 4.7244
  constraints: 1 centre point
  measures "d26" diameter of A0
extrude "Extrusion5" cut sketch "Sketch5" against normal blind 2.54
sketch "Sketch7" plane through (2, -2.54, -1.4) normal (0, -1, 0) x (1, 0, 0)
  point P0 (-2, 1.4)
sketch "Sketch8" plane through (2, -2.54, -1.4) normal (0, -1, 0) x (1, 0, 0)
  circle A0 centre (0, 0) radius 2.3622 projected
  circle A1 centre (0, 0) radius 4.8514
  point P0 (-2, 1.4)
  dimension "d35" = 9.7028
  constraints: 1 centre point, 1 coincident
  measures "d35" diameter of A1
extrude "Extrusion7" cut sketch "Sketch8" against normal blind 25.4
ref_plane "Work Plane3" through (16.975337, 38.1, 7.707365) normal (0.9981828, 0, -0.0602592) x (0, 1, 0)
sketch "Sketch9" plane through (16.975337, 38.1, 7.707365) normal (0.9981828, 0, -0.0602592) x (0, 1, 0)
  circle A0 centre (-1.85795, -0.008345) radius 1.3462
  point P0 (-38.1, -8.71628)
  dimension "d38" = 2.6924
  constraints: 1 centre point
  measures "d38" diameter of A0
extrude "Extrusion8" cut sketch "Sketch9" along normal mid plane 12.7
body "Solid1"
